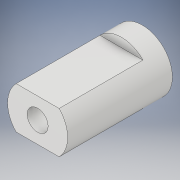
# Autodesk Inventor part: MotorShaft
Saved by Autodesk Inventor 2018 (Build 220112000, 112)
## iProperties
Created: 2018-01-12
Part Number: MotorShaft
Material: ABS Plastic
Document SubType Name: Modeling
Designer: Kyle
Density: 1.06 g/cm^3
Appearance: Smooth - White
Author: Kyle
Autodesk Inventor part; units mm, degrees
ref_plane "YZ Plane" through (0, 0, 0) normal (1, 0, 0) x (0, 1, 0)
ref_plane "XZ Plane" through (0, 0, 0) normal (0, 1, 0) x (-1, 0, 0)
ref_plane "XY Plane" through (0, 0, 0) normal (0, 0, 1) x (1, 0, 0)
sketch "Sketch1" plane through (0, 0, 0) normal (0, 0, 1) x (1, 0, 0)
  circle A0 centre (0, 0) radius 2.7305
  dimension "d0" = 5.461
  constraints: 1 centre point, 1 coincident
  measures "d0" diameter of A0
extrude "Extrusion1" add sketch "Sketch1" along normal blind 1.905
sketch "Sketch2" plane through (0, 0, 1.905) normal (0, 0, 1) x (1, 0, 0)
  circle A0 centre (0, 0) radius 2.7305 projected
  line L0 (-1.9562, 1.905) -> (1.9562, 1.905)
  line L1 (1.9562, -1.905) -> (-1.9562, -1.905)
  arc A1 (-1.9562, 1.905) -> (-1.9562, -1.905) centre (0, 0) ccw
  arc A2 (1.9562, -1.905) -> (1.9562, 1.905) centre (0, 0) ccw
  point P0 (0, 1.905)
  point P1 (0, -1.905)
  dimension "d3" = 1.905
  dimension "d4" = 1.905
  constraints: 5 point on circle, 4 end point, 2 centre point, 1 coincident, 1 horizontal, 1 parallel
  measures "d3" distance of point (0, 1.905) point (0, 0)
  measures "d4" distance of point (0, -1.905) point (0, 0)
extrude "Extrusion2" add sketch "Sketch2" along normal blind 7.62 contours A0 L1 L0
sketch "Sketch3" plane through (0, 0, 9.525) normal (0, 0, 1) x (1, 0, 0)
  circle A0 centre (0, 0) radius 2.7305 projected
  circle A1 centre (0, 0) radius 0.9525
  dimension "d7" = 1.905
  constraints: 1 centre point, 1 coincident
  measures "d7" diameter of A1
extrude "Extrusion3" cut sketch "Sketch3" against normal blind 7.62 contours A1
body "Solid1"
